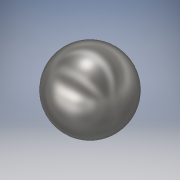
# Autodesk Inventor part: CasterBall
Saved by Autodesk Inventor 2018 (Build 220112000, 112)
## iProperties
Created: 2018-01-18
Part Number: CasterBall
Material: Stainless Steel
Document SubType Name: Modeling
Designer: mmarkle
Density: 8 g/cm^3
Appearance: Semi-Polished
Author: mmarkle
Autodesk Inventor part; units mm, degrees
ref_plane "YZ Plane" through (0, 0, 0) normal (1, 0, 0) x (0, 1, 0)
ref_plane "XZ Plane" through (0, 0, 0) normal (0, 1, 0) x (-1, 0, 0)
ref_plane "XY Plane" through (0, 0, 0) normal (0, 0, 1) x (1, 0, 0)
sketch "Sketch1" plane through (0, 0, 0) normal (0, 1, 0) x (-1, 0, 0)
  circle A0 centre (0, 0) radius 4.7625
  line L0 (-0.0627, -4.7621) -> (0.0627, 4.7621)
  dimension "d0" = 9.525
  constraints: 2 end point, 2 point on circle, 1 centre point, 1 coincident, 1 midpoint
  measures "d0" diameter of A0
revolve "Revolution1" add sketch "Sketch1" angle 360 about axis through (0.0627, 0, -4.7621) along (-0.0131568, 0, 0.9999134) picked at (0.3707, 1.5436) contours A0 L0
body "Solid1"
